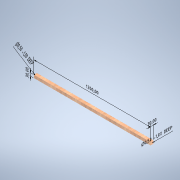
# Autodesk Inventor part: lange_Stange
Saved by Autodesk Inventor 2020.3 (Build 243373000, 373)
## iProperties
Created: 2020-09-30
Part Number: lange_Stange
Material: Birch
Document SubType Name: Modeling
Designer: Mara
Density: 0.512 g/cm^3
Appearance: Birch - Natural Medium Gloss
Author: Mara
Autodesk Inventor part; units mm, degrees
ref_plane "YZ Plane" through (0, 0, 0) normal (1, 0, 0) x (0, 1, 0)
ref_plane "XZ Plane" through (0, 0, 0) normal (0, 1, 0) x (-1, 0, 0)
ref_plane "XY Plane" through (0, 0, 0) normal (0, 0, 1) x (1, 0, 0)
sketch "Sketch1" plane through (0, 0, 0) normal (0, 0, 1) x (1, 0, 0)
  line L0 (-600, -15) -> (600, -15)
  line L1 (600, -15) -> (600, 15)
  line L2 (600, 15) -> (-600, 15)
  line L3 (-600, 15) -> (-600, -15)
  line L4 (-600, -15) -> (600, 15) construction
  line L5 (600, -15) -> (-600, 15) construction
  point P0 (0, 0)
  dimension "d0" = 1200
  dimension "d1" = 30
  constraints: 12 end point, 2 midpoint, 2 parallel, 1 horizontal, 1 perpendicular
  measures "d0" distance of L2.end L1.end
  measures "d1" distance of L1.end L0.end
extrude "Extrusion1" add sketch "Sketch1" along normal blind 30
sketch "Sketch2" plane through (600, -15, 0) normal (1, 0, 0) x (0, 0, -1)
  line L0 (0, 0) -> (0, 30) projected
  line L1 (0, 30) -> (-30, 30) projected
  line L2 (-30, 0) -> (-30, 30) projected
  line L3 (0, 0) -> (-30, 0) projected
  circle A0 centre (-15, 15) radius 15 construction
  circle A1 centre (-15, 15) radius 2.5
  point P0 (0, 15)
  dimension "d13" = 5
  constraints: 3 tangent, 2 centre point, 1 coincident
  measures "d13" diameter of A1
extrude "Extrusion2" cut sketch "Sketch2" against normal blind 10 contours A1
sketch "Sketch3" plane through (-600, -15, 0) normal (-1, 0, 0) x (0, 0, 1)
  circle A0 centre (15, 15) radius 2.5 projected
  point P0 (0, 15)
extrude "Extrusion3" cut sketch "Sketch3" against normal blind 10
body "Solid1"
